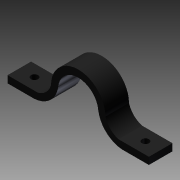
# Autodesk Inventor part: braket motor kipas
Saved by Autodesk Inventor 2012 (Build 160160000, 160)
## iProperties
Created: 2012-12-20
Part Number: braket motor kipas
Material: Default
Document SubType Name: Modeling
Designer: Irwan Haryanto
Density: 1 g/cm^3
Author: Irwan Haryanto
Autodesk Inventor part; units mm, degrees
ref_plane "YZ Plane" through (0, 0, 0) normal (1, 0, 0) x (0, 1, 0)
ref_plane "XZ Plane" through (0, 0, 0) normal (0, 1, 0) x (-1, 0, 0)
ref_plane "XY Plane" through (0, 0, 0) normal (0, 0, 1) x (1, 0, 0)
sketch "Sketch1" plane through (0, 0, 0) normal (0, 0, 1) x (1, 0, 0)
  arc A0 (8.5146, 0.7768) -> (-8.5146, 0.7768) centre (0, 0) ccw
  line L0 (-18.6378, -8.55) -> (-30, -8.55)
  line L1 (30, -8.55) -> (30, -5.55)
  line L2 (30, -5.55) -> (17.1, -5.55)
  line L3 (-30, -8.55) -> (-30, -5.55)
  line L4 (-30, -5.55) -> (-17.1, -5.55)
  arc A1 (11.55, 0) -> (17.1, -5.55) centre (19.2544, 2.1544) ccw
  line L5 (11.55, 0) -> (17.1, -5.55) construction
  line L6 (11.55, 0) -> (19.3989, 0) construction
  arc A2 (8.4438, 1.3433) -> (18.6378, -8.55) centre (19.3906, 2.4242) ccw
  arc A3 (-17.1, -5.55) -> (-11.55, 0) centre (-19.2544, 2.1544) ccw
  arc A4 (-18.6378, -8.55) -> (-8.4438, 1.3433) centre (-19.3906, 2.4242) ccw
  line L7 (18.6378, -8.55) -> (30, -8.55)
  arc A5 (11.55, 0) -> (-11.55, 0) centre (0, 0) ccw
  dimension "d0" = 17.1
  dimension "d3" = 3
  dimension "d6" = 45
  dimension "d7" = 8
  dimension "d8" = 11
  constraints: 16 end point, 15 point on circle, 6 centre point, 4 perpendicular, 2 horizontal, 2 tangent, 1 coincident, 1 collinear, 1 equal length
  measures "d0" diameter of A0
  measures "d3" distance of L1.start L1.end
  measures "d6" angle of L5 L6
  measures "d7" radius of A1
  measures "d8" radius of A2
extrude "Extrusion1" add sketch "Sketch1" against normal blind 10 contours A0 A4 L0 L3 L4 A3 A5 A1 L2 L1 L7 A2
sketch "Sketch2" plane through (17.1, -5.55, 0) normal (0, 1, 0) x (1, 0, 0)
  circle A0 centre (6.45, 5) radius 1.5
  point P0 (-17.1, 0)
  dimension "d11" = 3
  constraints: 1 centre point
  measures "d11" diameter of A0
hole "Hole1" at (23.55, -5.55, -5) direction (0, -1, 0) diameter 3 end through all
sketch "Sketch3" plane through (-30, -5.55, 0) normal (0, 1, 0) x (1, 0, 0)
  circle A0 centre (6.45, 5) radius 1.5
  point P0 (30, 0)
  dimension "d19" = 3
  constraints: 1 centre point
  measures "d19" diameter of A0
hole "Hole2" at (-23.55, -5.55, -5) direction (0, -1, 0) diameter 3 end through all
sketch "Sketch4" plane through (-30, -8.55, 0) normal (0, -1, 0) x (1, 0, 0)
  circle A0 centre (6.45, -5) radius 1.5 projected
  line L0 (0, -10) -> (11.3622, -10) projected
  line L1 (11.3622, 0) -> (11.3622, -10) projected
  line L2 (0, 0) -> (11.3622, 0) projected
  line L3 (0, 0) -> (0, -10) projected
  point P0 (30, 0)
body "Solid1"
